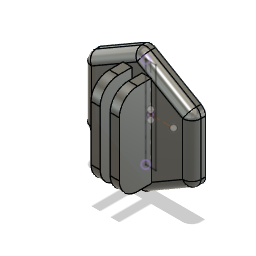
Hex Base Medium (Autodesk Fusion 360 design; units mm, degrees)
Autodesk Fusion 360 part; units mm, degrees
sketch "Sketch3" plane through (0, 0, 0) normal (0, 0, 1) x (1, 0, 0)
  line L0 (12, 6.9282) -> (0, 13.8564)
  line L1 (0, 13.8564) -> (-12, 6.9282)
  line L2 (-12, 6.9282) -> (-12, -6.9282)
  line L3 (-12, -6.9282) -> (0, -13.8564)
  line L4 (0, -13.8564) -> (12, -6.9282)
  line L5 (12, -6.9282) -> (12, 6.9282)
  line L6 (0, -13.8564) -> (0, 13.8564) construction
  dimension "d10" = 12
  constraint vertical L6
  measures "d10" distance of origin L5
extrude "Extrude2" add sketch "Sketch3" along normal blind 3
sketch "Sketch4" plane through (0, 0, 3) normal (0, 0, 1) x (1, 0, 0)
  line L0 (12, -6.9282) -> (12, 6.9282)
  line L1 (12, 6.9282) -> (0, 13.8564)
  line L2 (0, 13.8564) -> (-12, 6.9282)
  line L3 (-12, 6.9282) -> (-12, -6.9282)
  line L4 (-12, -6.9282) -> (0, -13.8564)
  line L5 (0, -13.8564) -> (12, -6.9282)
  line L6 (-3.1, 10) -> (-3.1, -10)
  line L7 (-3.1, -10) -> (-1.1, -10)
  line L8 (-1.1, -10) -> (-1.1, 10)
  line L9 (-1.1, 10) -> (-3.1, 10)
  line L10 (1.1, 10) -> (1.1, -10)
  line L11 (1.1, -10) -> (3.1, -10)
  line L12 (3.1, -10) -> (3.1, 10)
  line L13 (3.1, 10) -> (1.1, 10)
  line L14 (0, 14.3974) -> (0, -14) construction
  line L15 (-16.6832, 0) -> (20.9421, 0) construction
  dimension "d13" = 20
  dimension "d14" = 2
  dimension "d15" = 2.2
  constraint perpendicular L6 L7
  constraint parallel L6 L8
  constraint parallel L7 L9
  constraint perpendicular L10 L11
  constraint parallel L10 L12
  constraint parallel L11 L13
  constraint vertical L6
  constraint equal L6 L10
  constraint parallel L6 L10
  constraint equal L9 L13
  constraint collinear L9 L13
  constraint parallel L10 L14
  constraint symmetric L8 L10 L14
  constraint coincident origin L14
  constraint perpendicular L0 L15
  constraint coincident origin L15
  constraint symmetric L7 L9 L15
  measures "d13" distance of L6.start L6.end
  measures "d14" distance of L6.start L8.end
  measures "d15" distance of L8 L10
extrude "Extrude3" add sketch "Sketch4" along normal blind 7 contours L6 L7 L8 L9 | L10 L11 L12 L13
sketch "Sketch5" plane through (0, 0, 0) normal (0, 0, -1) x (-1, 0, 0)
  line L0 (-12, 6.9282) -> (-12, -6.9282)
  line L1 (-12, -6.9282) -> (0, -13.8564)
  line L2 (0, -13.8564) -> (12, -6.9282)
  line L3 (12, -6.9282) -> (12, 6.9282)
  line L4 (12, 6.9282) -> (0, 13.8564)
  line L5 (0, 13.8564) -> (-12, 6.9282)
  line L6 (-1.1, 10) -> (1.1, 10)
  line L7 (1.1, 10) -> (1.1, -10)
  line L8 (1.1, -10) -> (-1.1, -10)
  line L9 (-1.1, -10) -> (-1.1, 10)
  line L10 (0, 0) -> (-5, 0) construction
  line L11 (0, 10) -> (0, 0) construction
  line L12 (1.1, -10) -> (1.1, 10) construction
  line L13 (-1.1, 0) -> (1.1, 0) construction
  line L14 (0, 1) -> (0, -1) construction
  line L15 (0, 0) -> (0, -10) construction
  dimension "d18" = 20
  dimension "d19" = 2.2
  constraint horizontal L6
  constraint vertical L7
  constraint horizontal L8
  constraint vertical L9
  constraint perpendicular L8 L11
  constraint midpoint L8 L15.end
  constraint midpoint L6 L11.start
  constraint midpoint L9 L13.start
  constraint midpoint L7 L13.end
  constraint coincident L14 L10.start
  constraint coincident L13 L10.start
  constraint perpendicular L8 L15
  constraint coincident L10.start L11.end
  measures "d18" distance of L6.start L8.end
  measures "d19" distance of L6.start L6.end
extrude "Extrude4" cut sketch "Sketch5" against normal blind 2 contours L6 L7 L8 L9
fillet "Fillet1" radius 4 4 edges at (2.1, -10, 10) (-2.1, -10, 10) (2.1, 10, 10) (-2.1, 10, 10)
fillet "Fillet2" radius 2 6 edges at (12, -6.9282, 1.5) (0, -13.8564, 1.5) (-12, -6.9282, 1.5) (-12, 6.9282, 1.5) (12, 6.9282, 1.5) (0, 13.8564, 1.5)
fillet "Fillet3" radius 0.5 4 edges at (0, -10, 0) (-1.1, 0, 0) (0, 10, 0) (1.1, 0, 0)
fillet "Fillet5" radius 2 12 edges at (0, 13.547, 3) (-6, 10.3923, 3) (-11.7321, 6.7735, 3) (-12, 0, 3) (-11.7321, -6.7735, 3) (-6, -10.3923, 3) (0, -13.547, 3) (6, -10.3923, 3) (11.7321, -6.7735, 3) (12, 0, 3) (11.7321, 6.7735, 3) (6, 10.3923, 3)
named bodies: "Hex Base Medium"
